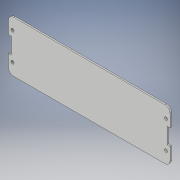
# Autodesk Inventor part: Plain Front Pannel
Saved by Autodesk Inventor 2019 (Build 230136000, 136)
## iProperties
Created: 2020-09-01
Part Number: Plain Front Pannel
Material: Generic
Document SubType Name: Modeling
Designer: johnh
Density: 1 g/cm^3
Appearance: Default
Author: johnh
Autodesk Inventor part; units mm, degrees
ref_plane "YZ Plane" through (0, 0, 0) normal (1, 0, 0) x (0, 1, 0)
ref_plane "XZ Plane" through (0, 0, 0) normal (0, 1, 0) x (-1, 0, 0)
ref_plane "XY Plane" through (0, 0, 0) normal (0, 0, 1) x (1, 0, 0)
sketch "Sketch1" plane through (0, 0, 0) normal (0, 0, 1) x (1, 0, 0)
  line L0 (0, 0) -> (201.5998, 0)
  line L1 (201.5998, 0) -> (201.5998, 63.754)
  line L2 (201.5998, 63.754) -> (0, 63.754)
  line L3 (0, 63.754) -> (0, 0)
  line L4 (0, 41.8592) -> (3.7465, 41.8592)
  line L5 (3.7465, 41.8592) -> (3.7465, 21.8948)
  line L6 (3.7465, 21.8948) -> (0, 21.8948)
  line L7 (0, 21.8948) -> (0, 41.8592)
  line L8 (201.5998, 41.8592) -> (197.8533, 41.8592)
  line L9 (197.8533, 41.8592) -> (197.8533, 21.8948)
  line L10 (197.8533, 21.8948) -> (201.5998, 21.8948)
  line L11 (201.5998, 21.8948) -> (201.5998, 41.8592)
  circle A0 centre (5.0546, 49.1744) radius 1.9558
  circle A1 centre (5.0546, 14.5796) radius 1.9558
  circle A2 centre (196.5452, 14.5796) radius 1.9558
  circle A3 centre (196.5452, 49.1744) radius 1.9558
  dimension "d0" = 201.5998
  dimension "d1" = 63.754
  dimension "d2" = 3.7465
  dimension "d3" = 19.9644
  dimension "d4" = 21.8948
  dimension "d6" = 3.7465
  dimension "d8" = 3.9116
  dimension "d9" = 12.6238
  dimension "d10" = 3.0988
  dimension "d11" = 3.9116
  dimension "d12" = 12.6238
  dimension "d13" = 3.0988
  dimension "d14" = 3.9116
  dimension "d15" = 3.0988
  constraints: 24 end point, 6 parallel, 4 centre point, 3 horizontal, 3 perpendicular, 2 point on line
  measures "d0" distance of L2.end L1.end
  measures "d1" distance of L1.end L0.end
  measures "d2" distance of L4.start L4.end
  measures "d3" distance of L4.end L5.end
  measures "d4" distance between parallel lines of L2 L4
  measures "d6" distance of L8.start L8.end
  measures "d8" diameter of A0
  measures "d9" distance edge to line of A0 L2
  measures "d10" distance edge to line of A0 L3
  measures "d11" diameter of A1
  measures "d12" distance edge to line of A1 L0
  measures "d13" distance edge to line of A1 L3
  measures "d14" diameter of A2
  measures "d15" distance edge to line of A2 L1
extrude "Extrusion1" add sketch "Sketch1" along normal blind 1.8796 contours L3 L6 L5 L4 L2 L1 L8 L9 L10 L0
fillet "Fillet1" radius 6.35 4 edges at (0, 63.754, 0.9398) (201.5998, 63.754, 0.9398) (201.5998, 0, 0.9398) (0, 0, 0.9398)
body "Solid1"
